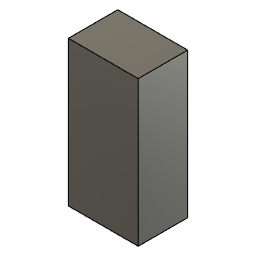
Suporte_Lipo_2 (Autodesk Fusion 360 archive; units mm, degrees)
design "Bateria_Lipo"
Autodesk Fusion 360 part; units mm, degrees
sketch "Sketch1" plane through (0, 0, 0) normal (0, 1, 0) x (1, 0, 0)
  line L0 (-32.5, 23) -> (32.5, 23)
  line L1 (32.5, 23) -> (32.5, -23)
  line L2 (32.5, -23) -> (-32.5, -23)
  line L3 (-32.5, -23) -> (-32.5, 23)
  line L4 (-32.5, 23) -> (32.5, -23) construction
  line L5 (32.5, 23) -> (-32.5, -23) construction
  dimension "d1" = 46
  dimension "d2" = 65
  constraint perpendicular L0 L1
  constraint parallel L0 L2
  constraint parallel L1 L3
  constraint horizontal L0
  constraint coincident L4 origin
  constraint coincident L5 origin
  measures "d1" distance of L0.start L2.end
  measures "d2" distance of L0.start L0.end
extrude "Extrude1" add sketch "Sketch1" along normal blind 135
